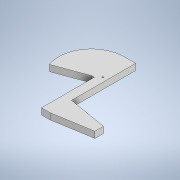
# Autodesk Inventor part: Mache à air
Saved by Autodesk Inventor 2020 (Build 240168000, 168)
## iProperties
Created: 2019-10-24
Part Number: Mache à air
Material: Générique
Document SubType Name: Modeling
Designer: erwan
Density: 1 g/cm^3
Appearance: Par défaut
Author: erwan
Autodesk Inventor part; units mm, degrees
ref_plane "YZ Plane" through (0, 0, 0) normal (1, 0, 0) x (0, 1, 0)
ref_plane "XZ Plane" through (0, 0, 0) normal (0, 1, 0) x (-1, 0, 0)
ref_plane "XY Plane" through (0, 0, 0) normal (0, 0, 1) x (1, 0, 0)
sketch "Esquisse1" plane through (0, 0, 0) normal (0, 1, 0) x (-1, 0, 0)
  line L0 (0, 0) -> (30, 0)
  line L1 (30, 0) -> (30, -185)
  line L2 (30, -185) -> (40, -185)
  line L3 (0, -300) -> (40, -300)
  arc A0 (40, -300) -> (148.0647, -145.6677) centre (40, -185) ccw
  line L4 (40, -185) -> (148.0647, -145.6677) construction
  line L5 (40, -185) -> (40, -300) construction
  line L6 (148.0647, -145.6677) -> (40, -185)
  line L7 (0, -300) -> (0, -75)
  line L8 (-135, -37.5) -> (-135, -52.5)
  line L9 (-135, -52.5) -> (0, -75)
  line L10 (-135, -37.5) -> (-135, -22.5)
  line L11 (-135, -22.5) -> (0, 0)
  circle A1 centre (15, -200) radius 2.5
  dimension "d1" = 30
  dimension "d2" = 185
  dimension "d3" = 10
  dimension "d4" = 110
  dimension "d5" = 115
  dimension "d6" = 225
  dimension "d11" = 135
  dimension "d12" = 30
  dimension "d13" = 22.5
  dimension "d14" = 22.5
  dimension "d16" = 5
  dimension "d17" = 100
  dimension "d18" = 15
  constraints: 24 end point, 3 horizontal, 3 vertical, 2 centre point, 2 point on circle, 1 coincident, 1 collinear, 1 point on line
  measures "d1" distance of L0.start L0.end
  measures "d2" distance of L0.end L1.end
  measures "d3" distance of L1.end L2.end
  measures "d4" angle of L5 L4
  measures "d5" radius of A0
  measures "d6" distance of L3.start L7.end
  measures "d11" horizontal distance of L8.end L7.end
  measures "d12" distance of L8.end L10.end
  measures "d13" vertical distance of L10.end L0.start
  measures "d14" vertical distance of L7.end L8.end
  measures "d16" diameter of A1
  measures "d17" distance from line of L3 A1.centre
  measures "d18" distance from line of L7 A1.centre
extrude "Extrusion1" add sketch "Esquisse1" along normal blind 22
